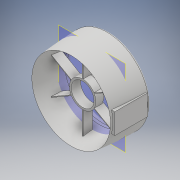
# Autodesk Inventor part: betterDuct
Saved by Autodesk Inventor 2018 (Build 220112000, 112)
## iProperties
Created: 2018-01-09
Part Number: betterDuct
Material: Generic
Document SubType Name: Modeling
Designer: mzhang
Density: 1 g/cm^3
Appearance: Default
Author: mzhang
Autodesk Inventor part; units mm, degrees
ref_plane "YZ Plane" through (0, 0, 0) normal (1, 0, 0) x (0, 1, 0)
ref_plane "XZ Plane" through (0, 0, 0) normal (0, 1, 0) x (-1, 0, 0)
ref_plane "XY Plane" through (0, 0, 0) normal (0, 0, 1) x (1, 0, 0)
sketch "Sketch2" plane through (0, 0, 0) normal (0, 0, 1) x (1, 0, 0)
  line L0 (0, 0) -> (37.25, 0)
  arc A0 (37.2924, 0.302) -> (37.2902, -0.2805) centre (39.27, 0.0031) ccw
  line L1 (0, 2.5402) -> (0, -5.2874)
  line L2 (37.27, 1.2556) -> (37.27, -1.8319)
  arc A1 (41.7179, 7.7108) -> (37.27, 1.2556) centre (44.178, 1.2556) ccw
  arc A2 (37.27, -1.8319) -> (41.8601, -32.1884) centre (125.7254, -3.9821) ccw
  arc A3 (44.2572, 5.9558) -> (41.7179, 7.7108) centre (42.3847, 5.9611) ccw
  arc A4 (41.8601, -32.1884) -> (44.2572, 5.9593) centre (-269.713, 6.5393) ccw
  point P0 (42.726, 0)
  dimension "d0" = 37.25
  constraints: 12 point on circle, 6 end point, 5 centre point, 2 tangent, 2 vertical, 1 horizontal
  measures "d0" distance of L0.start L0.end
revolve "Revolution1" add sketch "Sketch2" angle 360 about axis through (0, 2.5402, 0) along (0, -1, 0)
ref_plane "Work Plane1" through (0, -10, 0) normal (0, 1, 0) x (1, 0, 0)
sketch "Sketch4" plane through (0, -10, 0) normal (0, 1, 0) x (1, 0, 0)
  arc A0 (-33.3311, 19.6768) -> (-33.7061, 19.0272) centre (0, 0) ccw projected
  line L0 (-33.3311, 19.6768) -> (-12.0191, 7.3723) projected
  arc A1 (-0.375, 14.095) -> (-12.0191, 7.3723) centre (0, 0) ccw projected
  line L1 (-0.375, 14.095) -> (-0.375, 38.704) projected
  arc A2 (0.375, 38.704) -> (-0.375, 38.704) centre (0, 0) ccw projected
  line L2 (0.375, 38.704) -> (0.375, 14.095) projected
  arc A3 (12.0191, 7.3723) -> (0.375, 14.095) centre (0, 0) ccw projected
  line L3 (12.0191, 7.3723) -> (33.3311, 19.6768) projected
  arc A4 (33.7061, 19.0272) -> (33.3311, 19.6768) centre (0, 0) ccw projected
  line L4 (33.7061, 19.0272) -> (12.3941, 6.7227) projected
  arc A5 (12.3941, -6.7227) -> (12.3941, 6.7227) centre (0, 0) ccw projected
  line L5 (12.3941, -6.7227) -> (33.7061, -19.0272) projected
  arc A6 (33.3311, -19.6768) -> (33.7061, -19.0272) centre (0, 0) ccw projected
  line L6 (33.3311, -19.6768) -> (12.0191, -7.3723) projected
  arc A7 (0.375, -14.095) -> (12.0191, -7.3723) centre (0, 0) ccw projected
  line L7 (0.375, -14.095) -> (0.375, -38.704) projected
  arc A8 (-0.375, -38.704) -> (0.375, -38.704) centre (0, 0) ccw projected
  line L8 (-0.375, -38.704) -> (-0.375, -14.095) projected
  arc A9 (-12.0191, -7.3723) -> (-0.375, -14.095) centre (0, 0) ccw projected
  line L9 (-12.0191, -7.3723) -> (-33.3311, -19.6768) projected
  arc A10 (-33.7061, -19.0272) -> (-33.3311, -19.6768) centre (0, 0) ccw projected
  line L10 (-33.7061, -19.0272) -> (-12.3941, -6.7227) projected
  arc A11 (-12.3941, 6.7227) -> (-12.3941, -6.7227) centre (0, 0) ccw projected
  line L11 (-12.3941, 6.7227) -> (-33.7061, 19.0272) projected
  circle A12 centre (0, 0) radius 12.1 projected
extrude "Extrusion2" add sketch "Sketch4" against normal blind 10
sketch "Sketch5" plane through (0, -10, 0) normal (0, 1, 0) x (1, 0, 0)
  line L0 (42.4432, 11) -> (44.2578, 11)
  line L1 (44.2578, 11) -> (44.2578, -11)
  line L2 (44.2578, -11) -> (42.4432, -11)
  line L3 (42.4432, -11) -> (42.4432, 11)
  line L4 (42.4432, 11) -> (44.2578, -11) construction
  line L5 (44.2578, 11) -> (42.4432, -11) construction
  point P0 (0, 0)
  point P1 (43.3505, 0)
  dimension "d16" = 22
  constraints: 12 end point, 2 midpoint, 2 parallel, 1 horizontal, 1 perpendicular
  measures "d16" distance of L0.end L1.end
extrude "Extrusion3" add sketch "Sketch5" along normal blind 15 and the other way blind 20
sketch "Sketch6" plane through (0, -30, 0) normal (0, -1, 0) x (1, 0, 0)
  circle A0 centre (0, 0) radius 41.8601 projected
  line L0 (42.4432, 11) -> (40.389, 11)
  line L1 (42.4432, -11) -> (40.389, -11)
  line L2 (42.4432, 11) -> (42.4432, -11) projected
  line L3 (42.4432, -11) -> (42.4432, 11)
  constraints: 6 end point, 2 point on circle, 1 horizontal, 1 vertical
extrude "Extrusion4" add sketch "Sketch6" against normal up to surface (35 mm away) contours A0 L0 L2 L1
fillet "Fillet1" radius 2 6 edges at (-7.05, -10, 12.211) (-14.1, -10, 0) (-7.05, -10, -12.211) (7.05, -10, -12.211) (14.1, -10, 0) (7.05, -10, 12.211)
body "Solid1"
